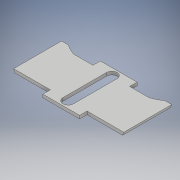
# Autodesk Inventor part: Deslizador
Saved by Autodesk Inventor 2017 (Build 210142000, 142)
## iProperties
Created: 2017-01-19
Part Number: Deslizador
Material: Generic
Document SubType Name: Modeling
Designer: A. Matías Quezada
Density: 1 g/cm^3
Appearance: Default
Author: A. Matías Quezada
Autodesk Inventor part; units mm, degrees
ref_plane "YZ Plane" through (0, 0, 0) normal (1, 0, 0) x (0, 1, 0)
ref_plane "XZ Plane" through (0, 0, 0) normal (0, 1, 0) x (-1, 0, 0)
ref_plane "XY Plane" through (0, 0, 0) normal (0, 0, 1) x (1, 0, 0)
sketch "Sketch1" plane through (0, 0, 0) normal (0, 0, 1) x (1, 0, 0)
  line L0 (0, 0) -> (0, 45)
  line L1 (0, 45) -> (-6.5, 45)
  line L2 (0, 0) -> (-34.5, 0)
  line L3 (-34.5, 0) -> (-34.5, -7)
  line L4 (-34.5, -7) -> (-51.75, -7)
  line L5 (-51.75, -7) -> (-51.75, 47)
  line L6 (-51.75, 47) -> (-34.5, 47)
  line L7 (-34.5, 47) -> (-34.5, 40)
  line L8 (-34.5, 40) -> (-16.5, 40)
  arc A0 (-16.5, 40) -> (-6.5, 45) centre (-24.6814, 68.8629) ccw
  line L9 (-103.5, 0) -> (-103.5, 45)
  line L10 (-103.5, 45) -> (-97, 45)
  line L11 (-103.5, 0) -> (-69, 0)
  line L12 (-69, 0) -> (-69, -7)
  line L13 (-69, -7) -> (-51.75, -7)
  line L14 (-51.75, 47) -> (-69, 47)
  line L15 (-69, 47) -> (-69, 40)
  line L16 (-69, 40) -> (-87, 40)
  arc A1 (-97, 45) -> (-87, 40) centre (-78.8186, 68.8629) ccw
  dimension "d16" = 10
  dimension "d17" = 30
  dimension "d18" = 6.5
  dimension "d19" = 5
  dimension "d20" = 40
  dimension "d23" = 34.5
  dimension "d24" = 103.5
  dimension "d25" = 54
  constraints: 34 end point, 9 symmetric about line, 7 perpendicular, 4 point on circle, 2 centre point, 2 equal length, 1 horizontal, 1 vertical, 1 other
  measures "d16" horizontal distance of L1.end L8.end
  measures "d17" radius of A0
  measures "d18" distance of L0.end L1.end
  measures "d19" distance between parallel lines of L1 L8
  measures "d20" distance between parallel lines of L11 L16
  measures "d23" distance between parallel lines of L7 L15
  measures "d24" distance between parallel lines of L0 L9
  measures "d25" distance between parallel lines of L13 L14
extrude "Body" add sketch "Sketch1" along normal blind 3
sketch "Sketch2" plane through (0, 0, 3) normal (0, 0, 1) x (1, 0, 0)
  line L0 (-56.75, -0.5) -> (-56.75, 40.5)
  arc A0 (-46.75, 40.5) -> (-56.75, 40.5) centre (-51.75, 40.5) ccw
  line L1 (-46.75, 40.5) -> (-46.75, -0.5)
  arc A1 (-56.75, -0.5) -> (-46.75, -0.5) centre (-51.75, -0.5) ccw
  line L2 (-16.5, 40) -> (-34.5, 40) projected
  line L3 (0, 0) -> (0, 45) projected
  line L4 (-34.5, -7) -> (-34.5, 0) projected
  line L5 (-34.5, 40) -> (-34.5, 0)
  line L6 (-131.212, 20) -> (6.3115, 20)
  point P0 (-46.75, 20)
  point P1 (-34.5, 20)
  dimension "d28" = 41
  dimension "d30" = 46.75
  dimension "d31" = 10
  constraints: 8 end point, 4 point on circle, 4 tangent, 2 centre point, 2 midpoint, 2 point on line, 2 vertical, 1 collinear, 1 horizontal
  measures "d28" distance of A0.centre A1.centre
  measures "d30" distance between parallel lines of L3 L1
  measures "d31" distance between parallel lines of L1 L0
extrude "Extrusion2" cut sketch "Sketch2" against normal through all
draft "FaceDraft1" angle -20 pull direction (0, 0, 1) faces at (0, 15, 1) fixed edges at (0, 22.5, 3)
draft "FaceDraft2" angle -20 pull direction (0, 0, 1) faces at (-103.5, 30, 1) fixed edges at (-103.5, 22.5, 3)
equation "\"d16\" = deslizador_interruptor_largo"
equation "\"d17\" = deslizador_interruptor_angulo"
equation "\"d18\" = deslizador_interruptor_separacion"
equation "\"d19\" = deslizador_interruptor_ancho"
equation "\"d20\" = deslizador_ancho"
equation "\"d23\" = deslizador_apoyo_largo"
equation "\"d24\" = deslizador_largo"
equation "\"d25\" = deslizador_ancho + 2 * deslizador_apoyo_ancho"
equation "\"d26\" = deslizador_grosor"
equation "\"d28\" = deslizador_eje_movimiento"
equation "\"d30\" = deslizador_eje_separacion"
equation "\"d31\" = deslizador_eje_ancho"
equation "\"d34\" = tirador_deslizador_agarre"
equation "\"d35\" = tirador_deslizador_agarre"
equation "\"deslizador_interruptor_largo\" = 10"
equation "\"deslizador_interruptor_angulo\" = 30"
equation "\"deslizador_interruptor_separacion\" = 6.5"
equation "\"deslizador_interruptor_ancho\" = 5"
equation "\"deslizador_ancho\" = 40"
equation "\"deslizador_apoyo_largo\" = 34.5"
equation "\"deslizador_largo\" = 103.5"
equation "\"deslizador_apoyo_ancho\" = 7"
equation "\"deslizador_grosor\" = 3"
equation "\"deslizador_eje_movimiento\" = 41"
equation "\"deslizador_eje_separacion\" = 46.75"
equation "\"deslizador_eje_ancho\" = 10"
equation "\"tirador_deslizador_agarre\" = -20deg"
body "Solid1"
